Foehn_Adapter_v4 (Autodesk Fusion 360 design; units mm, degrees)
Autodesk Fusion 360 part; units mm, degrees
cylinder "CylinderPrimitive1" add diameter 38.5 height 10 placed x (1, 0, 0) y (0, 0, -1) z (0, 1, 0) at (0, 0, 0) makes body 1
extrude "Extrude1" cut 1 faces at (0.4795, 10, -5.5475) along direction (0, -1, 0) blind 5 on bodies 1 bodies 1
sketch "Sketch2" plane through (0, 0, 0) normal (1, 0, 0) x (0, 0, -1)
  line L0 (-19.25, 0) -> (-19.25, 2)
  line L1 (-19.25, 2) -> (-20, 2)
  line L2 (-19.25, 2) -> (-19.25, 2.5)
  line L3 (-19.25, 2.5) -> (-20, 2)
  line L4 (-19.25, 0) -> (-20, 2)
  dimension "d5" = 0.75
  constraint vertical L0
  constraint perpendicular L0 L1
  constraint perpendicular L1 L2
  measures "d5" distance of L0.end L1.end
revolve "Revolve1" add sketch "Sketch2" angle 100 about axis through (0, 1.75, 0) along (0, 1, 0) separate body makes body 2
copy_body "CopyPasteBodies1" bodies 2 makes body 3
move_body "Move1" bodies 3 to x (-1, 0, 0) y (0, 1, 0) z (0, 0, -1) at (0, 0, 0)
cylinder "CylinderPrimitive2" add diameter 55 height 5 placed x (1, 0, 0) y (0, 0, -1) z (0, 1, 0) at (0, 5, 0) bodies 1
cylinder "CylinderPrimitive3" cut diameter 34 height -16 placed x (1, 0, 0) y (0, 0, -1) z (0, 1, 0) at (0, 10, 0) bodies 1
cylinder "CylinderPrimitive4" cut diameter 48.2 height -4 placed x (1, 0, 0) y (0, 0, -1) z (0, 1, 0) at (0, 10, 0) bodies 1
sketch "Sketch7" plane through (0, 0, 0) normal (0, 0, 1) x (1, 0, 0)
  circle A0 through (-24.1, 10, 0) (12.05, 10, 20.8712) (12.05, 10, -20.8712)
  line L0 (23.9747, 10, -2.454) -> (23.9747, 8.5, -2.454)
  line L1 (24, 8.5) -> (25, 8.5)
  line L2 (24, 10) -> (25, 8.5)
  line L3 (24, 8.5) -> (24, 6)
  line L4 (24, 6) -> (25, 8.5)
  dimension "d13" = 1.5
  dimension "d14" = 1
  constraint horizontal L1
  constraint perpendicular L1 L3
  measures "d14" distance of L1.start L1.end
revolve "Revolve2" cut sketch "Sketch7" angle 360 about axis through (0, 1.75, 0) along (0, 1, 0) bodies 1
fillet "Fillet1" radius 0.1 7 edges at (-8.7149, 8.5, 22.4691) (-8.7149, 10, 22.4691) (-25.639, 10, 9.9444) (-25.639, 5, -9.9444) (-17.9473, 0, -6.9611) (6.1475, 0, 15.8496) (6.1475, 6, 15.8496) on bodies 1
delete_face "DeleteFace1" 1 faces at (-2.392, 0.05, -19.0873) on bodies 1
fillet "Fillet2" radius 0.5 1 edges at (-17.9473, 5, -6.9611) on bodies 1
combine "Combine1" operation add target body 1 tool bodies 2 3
delete_face "DeleteFace2" 1 faces at (-21.4904, 9.9866, 11.0175) on bodies 1
move_face "OffsetFaces1" offset -0.15 1 faces at (-9.3613, 9.5333, -22.2076) on bodies 1
fillet "Fillet3" radius 0.2 1 edges at (8.7692, 10, 22.6089) on bodies 1
move_face "OffsetFaces2" offset 0.23 1 faces at (2.3301, 2.3333, -19.1085) on bodies 1
sketch "Sketch8" plane through (0, 0, 0) normal (1, 0, 0) x (0, 0, -1)
  line L0 (-19.4, 0) -> (-20.7, 2)
  line L1 (-20.7, 2) -> (-19.4, 2.5)
  line L2 (-19.4, 2.5) -> (-19.4, 0)
  line L3 (-20.7, 2) -> (-19.4, 2)
  constraint vertical L2
  constraint coincident L2 L3.end
  constraint perpendicular L2 L3
revolve "Revolve3" add sketch "Sketch8" angle 120 about axis through (0, 1.75, 0) along (0, 1, 0) separate body makes body 4
copy_body "CopyPasteBodies2" bodies 4 makes body 5
move_body "Move2" bodies 5 to x (-1, 0, 0) y (0, 1, 0) z (0, 0, -1) at (0, 0, 0)
